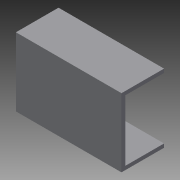
# Autodesk Inventor part: mount pour oeil
Saved by Autodesk Inventor 2014 (Build 180170000, 170)
## iProperties
Created: 2016-11-02
Part Number: mount pour oeil
Material: Générique
Document SubType Name: Modeling
Designer: 0034348
Density: 1 g/cm^3
Appearance: Par défaut
Author: 0034348
Autodesk Inventor part; units mm, degrees
ref_plane "YZ Plane" through (0, 0, 0) normal (1, 0, 0) x (0, 1, 0)
ref_plane "XZ Plane" through (0, 0, 0) normal (0, 1, 0) x (-1, 0, 0)
ref_plane "XY Plane" through (0, 0, 0) normal (0, 0, 1) x (1, 0, 0)
sketch "Esquisse1" plane through (0, 0, 0) normal (0, 1, 0) x (-1, 0, 0)
  line L0 (28.5, 18.5) -> (-28.5, 18.5)
  line L1 (-28.5, 18.5) -> (-28.5, -18.5)
  line L2 (-28.5, -18.5) -> (28.5, -18.5)
  line L3 (28.5, -18.5) -> (28.5, 18.5)
  line L4 (28.5, 18.5) -> (-28.5, -18.5) construction
  line L5 (-28.5, 18.5) -> (28.5, -18.5) construction
  point P0 (0, 0)
  dimension "d0" = 57
  dimension "d1" = 37
  constraints: 12 end point, 2 midpoint, 2 parallel, 1 horizontal, 1 perpendicular
  measures "d0" distance of L2.end L1.end
  measures "d1" distance of L1.end L0.end
extrude "Extrusion1" add sketch "Esquisse1" along normal blind 23
sketch "Esquisse2" plane through (0, 23, 0) normal (0, 1, 0) x (1, 0, 0)
  line L0 (-28.5, -18.5) -> (28.5, -18.5) projected
  line L1 (28.5, -18.5) -> (28.5, 18.5) projected
  line L2 (-28.5, 18.5) -> (-8.5, 18.5)
  line L3 (-8.5, 18.5) -> (-8.5, -18.5)
  line L4 (-8.5, -18.5) -> (-28.5, -18.5)
  line L5 (-28.5, -18.5) -> (-28.5, 18.5)
  line L6 (28.5, 18.5) -> (28.5, 16.5) construction
  line L7 (28.5, -18.5) -> (28.5, -16.5) construction
  line L8 (28.5, 16.5) -> (-8.5, 16.5)
  line L9 (-8.5, 16.5) -> (-8.5, -16.5)
  line L10 (-8.5, -16.5) -> (28.5, -16.5)
  line L11 (28.5, -16.5) -> (28.5, 16.5)
  point P0 (0, 0)
  dimension "d4" = 20
  dimension "d5" = 2
  dimension "d6" = 2
  dimension "d7" = 33
  constraints: 20 end point, 4 parallel, 4 point on line, 2 horizontal, 2 perpendicular
  measures "d4" distance of L3.end L4.end
  measures "d5" distance of L1.end L6.end
  measures "d6" distance of L0.end L7.end
  measures "d7" distance of L9.end L8.end
extrude "Extrusion2" cut sketch "Esquisse2" against normal blind 21 contours L3 L8 L1 L10
sketch "Esquisse3" plane through (-8.5, 23, 16.5) normal (1, 0, 0) x (0, 0, -1)
  line L0 (0, 0) -> (0, -21) projected
  line L1 (33, -21) -> (0, -21)
  line L2 (0, -21) -> (0, -2)
  line L3 (0, -2) -> (33, -2)
  line L4 (33, -2) -> (33, -21)
  point P0 (16.5, -23)
  dimension "d10" = 19
  constraints: 8 end point, 2 parallel, 1 horizontal, 1 perpendicular, 1 point on line
  measures "d10" distance of L1.end L2.end
extrude "Extrusion3" cut sketch "Esquisse3" against normal blind 18
sketch "Esquisse4" plane through (-28.5, 0, -18.5) normal (-1, 0, 0) x (0, 0, 1)
  line L0 (37, 0) -> (18.5, 0) construction
  line L1 (18.5, 0) -> (18.5, 11.5) construction
  line L2 (18.5, 11.5) -> (37, 11.5) construction
  line L3 (37, 11.5) -> (37, 0) construction
  line L4 (6.5, 4.25) -> (30.5, 4.25)
  line L5 (30.5, 4.25) -> (30.5, 18.75)
  line L6 (30.5, 18.75) -> (6.5, 18.75)
  line L7 (6.5, 18.75) -> (6.5, 4.25)
  line L8 (6.5, 4.25) -> (30.5, 18.75) construction
  line L9 (30.5, 4.25) -> (6.5, 18.75) construction
  dimension "d13" = 18.5
  dimension "d14" = 11.5
  dimension "d15" = 24
  dimension "d16" = 14.5
  constraints: 20 end point, 4 parallel, 2 horizontal, 2 midpoint, 2 perpendicular
  measures "d13" distance of L1.end L2.end
  measures "d14" distance of L0.end L1.end
  measures "d15" distance of L6.end L5.end
  measures "d16" distance of L5.end L4.end
extrude "Extrusion4" cut sketch "Esquisse4" against normal blind 5
